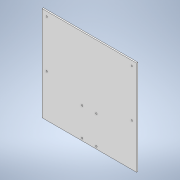
# Autodesk Inventor part: brackert-temporary-2
Saved by Autodesk Inventor 2021 (Build 250183000, 183)
## iProperties
Created: 2024-04-05
Part Number: brackert-temporary-2
Material: PC/ABS Plastic
Document SubType Name: Modeling
Designer: ASUS
Density: 0.357273 g/cm^3
Appearance: White
Author: ASUS
Autodesk Inventor part; units mm, degrees
ref_plane "YZ Plane" through (0, 0, 0) normal (1, 0, 0) x (0, 1, 0)
ref_plane "XZ Plane" through (0, 0, 0) normal (0, 1, 0) x (-1, 0, 0)
ref_plane "XY Plane" through (0, 0, 0) normal (0, 0, 1) x (1, 0, 0)
sketch "Sketch1" plane through (0, 0, 0) normal (0, 0, 1) x (1, 0, 0)
  line L0 (0, 0) -> (200, 0)
  line L1 (200, 0) -> (200, 200)
  line L2 (200, 200) -> (0, 200)
  line L3 (0, 200) -> (0, 0)
  circle A0 centre (85, 5) radius 1.5
  circle A1 centre (115, 5) radius 1.5
  circle A2 centre (85, 65) radius 1.5
  circle A3 centre (115, 65) radius 1.5
  circle A4 centre (10, 190) radius 1.5
  circle A5 centre (190, 190) radius 1.5
  circle A6 centre (10, 90) radius 1.5
  circle A7 centre (190, 90) radius 1.5
  dimension "d0" = 200
  dimension "d1" = 200
  dimension "d2" = 3
  dimension "d3" = 3
  dimension "d4" = 5
  dimension "d5" = 5
  dimension "d6" = 30
  dimension "d7" = 85
  dimension "d8" = 3
  dimension "d9" = 3
  dimension "d10" = 85
  dimension "d11" = 60
  dimension "d12" = 30
  dimension "d13" = 60
  dimension "d14" = 3
  dimension "d15" = 3
  dimension "d16" = 10
  dimension "d17" = 10
  dimension "d18" = 10
  dimension "d19" = 10
  dimension "d20" = 3
  dimension "d21" = 3
  dimension "d22" = 10
  dimension "d23" = 10
  dimension "d24" = 100
  dimension "d25" = 100
  constraints: 8 centre point, 8 end point, 2 parallel, 1 horizontal, 1 perpendicular
  measures "d0" distance between parallel lines of L0 L2
  measures "d1" distance between parallel lines of L1 L3
  measures "d2" diameter of A0
  measures "d3" diameter of A1
  measures "d4" distance from line of L0 A0.centre
  measures "d5" distance from line of L0 A1.centre
  measures "d6" distance of A1.centre A0.centre
  measures "d7" distance from line of L3 A0.centre
  measures "d8" diameter of A2
  measures "d9" diameter of A3
  measures "d10" distance from line of L3 A2.centre
  measures "d11" distance of A0.centre A2.centre
  measures "d12" distance of A2.centre A3.centre
  measures "d13" distance of A1.centre A3.centre
  measures "d14" diameter of A4
  measures "d15" diameter of A5
  measures "d16" distance from line of L3 A4.centre
  measures "d17" distance from line of L2 A4.centre
  measures "d18" distance from line of L1 A5.centre
  measures "d19" distance from line of L2 A5.centre
  measures "d20" diameter of A6
  measures "d21" diameter of A7
  measures "d22" distance from line of L3 A6.centre
  measures "d23" distance from line of L1 A7.centre
  measures "d24" distance of A6.centre A4.centre
  measures "d25" distance of A5.centre A7.centre
extrude "Extrusion1" add sketch "Sketch1" along normal blind 3
body "Solid1"
